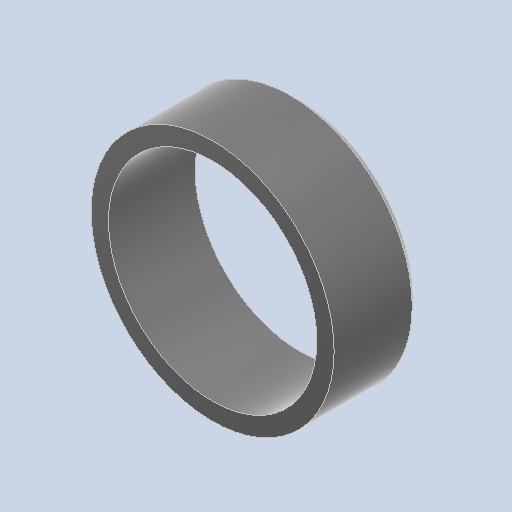
# Autodesk Inventor part: w5f12-14n
Saved by Autodesk Inventor 2023 (Build 270158000, 158)
## iProperties
Created: 2022-01-09
Part Number: w5f12-14n
Material: アセタール樹脂、黒
Document SubType Name: Modeling
Designer: acps
Density: 1.425 g/cm^3
Appearance: 滑らか - 黒
Mass: 0.283342 g
Surface Area: 4.76881 cm^2
Volume: 0.198837 cm^3
Author: acps
Autodesk Inventor part; units mm, degrees
ref_plane "YZ Plane" through (0, 0, 0) normal (1, 0, 0) x (0, 1, 0)
ref_plane "XZ Plane" through (0, 0, 0) normal (0, 1, 0) x (-1, 0, 0)
ref_plane "XY Plane" through (0, 0, 0) normal (0, 0, 1) x (1, 0, 0)
sketch "Sketch1" plane through (0, 0, 0) normal (0, 0, 1) x (1, 0, 0)
  circle A0 centre (0, 0) radius 6
  circle A1 centre (0, 0) radius 7
  dimension "d0" = 12
  dimension "d1" = 14
  constraints: 2 centre point, 2 coincident
  measures "d0" diameter of A0
  measures "d1" diameter of A1
extrude "Extrusion1" add sketch "Sketch1" against normal blind 5
chamfer "Chamfer1" distance 0.5 angle 45 1 edges at (-7, 0, -5)
body "Solid1"
